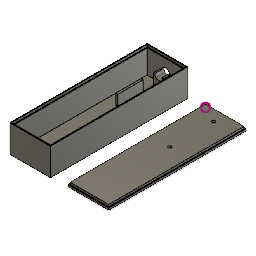
test v3-ok v1 v5 (Autodesk Fusion 360 design; units mm, degrees)
Autodesk Fusion 360 part; units mm, degrees
note: some values were not read from the file. Set by a fixed rule: which face or edge a step refers to.
sketch "スケッチ1" plane through (0, 0, 0) normal (0, 1, 0) x (1, 0, 0)
  line L0 (-40, 10) -> (0, 10)
  line L1 (0, 10) -> (0, -125)
  line L2 (0, -125) -> (-40, -125)
  line L3 (-40, -125) -> (-40, 10)
  line L4 (-31.0482, -10.0567) -> (-29.0482, -10.0567)
  line L5 (-29.0482, -10.0567) -> (-29.0482, -35.0567)
  line L6 (-29.0482, -35.0567) -> (-31.0482, -35.0567)
  line L7 (-31.0482, -35.0567) -> (-31.0482, -10.0567)
  line L8 (-40, -125) -> (-30, -125)
  line L9 (-40, -35) -> (-40, -125)
  line L10 (-40, 10) -> (0, 10)
  line L11 (0, 10) -> (0, 8)
  line L12 (0, 8) -> (-40, 8)
  line L13 (-40, 8) -> (-40, 10)
  line L14 (-40, 10) -> (-38, 10)
  line L15 (-38, 10) -> (-38, -125)
  line L16 (-38, -125) -> (-40, -125)
  line L17 (-40, -125) -> (-40, 10)
  line L18 (0, 10) -> (-2, 10)
  line L19 (-2, 10) -> (-2, -125)
  line L20 (-2, -125) -> (0, -125)
  line L21 (0, -125) -> (0, 10)
  line L22 (-40, -125) -> (0, -125)
  line L23 (0, -125) -> (0, -123)
  line L24 (0, -123) -> (-40, -123)
  line L25 (-40, -123) -> (-40, -125)
  dimension "d1" = 40
  dimension "d2" = 135
  dimension "d3" = 2
  dimension "d4" = 25
  dimension "d5" = 10
  dimension "d6" = 90
  dimension "d7" = 2
  dimension "d8" = 2
  dimension "d9" = 135
  dimension "d10" = 2
  dimension "d11" = 135
  dimension "d12" = 40
  dimension "d13" = 2
  measures "d2" distance of origin
  measures "d4" distance of origin
  measures "d9" distance of origin
  measures "d11" distance of origin
extrude "押し出し1" add sketch "スケッチ1" along normal blind 25 contours L0 L3 L10 L12 L13 L14 L15 L17 | L0 L10 L12 L15 L19 | L3 L9 L12 L15 L17 L24 | L0 L1 L10 L11 L12 L18 L19 L21 | L1 L12 L19 L21 L24 | L2 L8 L15 L19 L22 L24 | L2 L3 L8 L9 L15 L16 L17 L22 L24 L25 | L1 L2 L19 L20 L21 L22 L23 L24 makes body 1
sketch "スケッチ2" plane through (0, 0, 125) normal (0, 0, 1) x (1, 0, 0)
  line L0 (-40, 0) -> (0, 0)
  line L1 (0, 0) -> (0, 25)
  line L2 (0, 25) -> (-40, 25)
  line L3 (-40, 25) -> (-40, 0)
  line L4 (-40, 0) -> (0, 0)
  line L5 (0, 0) -> (0, -2)
  line L6 (0, -2) -> (-40, -2)
  line L7 (-40, -2) -> (-40, 0)
  dimension "d16" = 40
  dimension "d17" = 2
  measures "d17" distance of L0.end
extrude "押し出し2" add sketch "スケッチ2" against normal blind 135 contours L0 L4 L5 L6 L7 bodies 1
sketch "スケッチ3" plane through (0, 0, 0) normal (0, 1, 0) x (1, 0, 0)
  line L0 (-38, -123) -> (-28, -123)
  line L1 (-28, -123) -> (-28, -33)
  line L2 (-28, -33) -> (-38, -33)
  line L3 (-38, -33) -> (-38, -123)
  line L4 (-28, -33) -> (-26, -33)
  line L5 (-26, -33) -> (-26, -8)
  line L6 (-26, -8) -> (-28, -8)
  line L7 (-28, -8) -> (-28, -33)
  dimension "d20" = 90
  dimension "d21" = 10
  dimension "d22" = 25
  dimension "d23" = 2
  measures "d22" distance of origin
extrude "押し出し3" add sketch "スケッチ3" along normal blind 10 contours L4 L5 L6 L7 bodies 1
hole "穴1" at (-20, 11.5, -10) direction (0, 0, 1) diameter 7 depth 15 tip angle 118 bodies 1
sketch "スケッチ4" plane through (0, 0, -10) normal (0, 0, -1) x (-1, 0, 0)
  circle A0 centre (20, 11.5) radius 3.5
  line L0 (40, -2) -> (40, 25)
  line L1 (40, 25) -> (0, 25)
  line L2 (0, 25) -> (0, -2)
  line L3 (0, -2) -> (40, -2)
sketch "スケッチ5" plane through (0, 0, 0) normal (0, 1, 0) x (1, 0, 0)
  line L0 (-24.8616, 8) -> (-15, 8)
  line L1 (-15, 8) -> (-15, -2)
  line L2 (-15, -2) -> (-24.8616, -2)
  line L3 (-24.8616, -2) -> (-24.8616, 8)
  line L4 (-38, 8) -> (-2, 8)
extrude "押し出し4" add sketch "スケッチ5" along normal blind 15 separate body makes body 2
extrude "押し出し5" add 1 faces at (-21.5744, 15, -4.6667) along direction (0, 1, 0) blind 7 on bodies 2 bodies 2 1
extrude "押し出し6" cut sketch "スケッチ4" against normal blind 34 contours A0 bodies 2
extrude "押し出し7" cut 1 faces at (-21.5744, 22, -4.6667) along direction (0, -1, 0) blind 10 on bodies 2 bodies 2
move_face "面をオフセット1" offset -3 1 faces at (-19.8703, 2.6697, 2) on bodies 2
sketch "スケッチ6" plane through (0, 25, 0) normal (0, 1, 0) x (-1, 0, 0)
  line L0 (38, 123) -> (38, -8)
  line L1 (38, -8) -> (2, -8)
  line L2 (2, -8) -> (2, 123)
  line L3 (2, 123) -> (38, 123)
  line L4 (40, -10) -> (40, 125)
  line L5 (40, 125) -> (0, 125)
  line L6 (0, 125) -> (0, -10)
  line L7 (0, -10) -> (40, -10)
  line L8 (39, -9) -> (1, -9)
  line L9 (1, -9) -> (1, 124)
  line L10 (1, 124) -> (39, 124)
  line L11 (39, 124) -> (39, -9)
  dimension "d38" = 133
  measures "d38" distance of origin
extrude "押し出し8" cut sketch "スケッチ6" against normal blind 2 contours L8 L9 L10 L11 bodies 2
sketch "スケッチ7" plane through (0, 0, 0) normal (0, 1, 0) x (1, 0, 0)
  line L0 (18.1709, 9.0329) -> (58.1709, 9.0329)
  line L1 (58.1709, 9.0329) -> (58.1709, -125.9671)
  line L2 (58.1709, -125.9671) -> (18.1709, -125.9671)
  line L3 (18.1709, -125.9671) -> (18.1709, 9.0329)
  dimension "d41" = 135
  dimension "d42" = 40
extrude "押し出し9" add sketch "スケッチ7" along normal blind 2 separate body makes body 3
sketch "スケッチ8" plane through (0, 0, 0) normal (0, 1, 0) x (1, 0, 0)
sketch "スケッチ9" plane through (0, 2, 0) normal (0, 1, 0) x (-1, 0, 0)
  line L0 (-18.1709, 125.9671) -> (-58.1709, 125.9671)
  line L1 (-58.1709, 125.9671) -> (-58.1709, -9.0329)
  line L2 (-58.1709, -9.0329) -> (-18.1709, -9.0329)
  line L3 (-18.1709, -9.0329) -> (-18.1709, 125.9671)
  line L4 (-18.1709, -9.0329) -> (-19.1709, -9.0329)
  line L5 (-19.1709, -9.0329) -> (-19.1709, -8.0329)
  line L6 (-19.1709, -8.0329) -> (-18.1709, -8.0329)
  line L7 (-18.1709, -8.0329) -> (-18.1709, -9.0329)
  line L8 (-19.1709, -8.0329) -> (-57.1709, -8.0329)
  line L9 (-57.1709, -8.0329) -> (-57.1709, 124.9671)
  line L10 (-57.1709, 124.9671) -> (-19.1709, 124.9671)
  line L11 (-19.1709, 124.9671) -> (-19.1709, -8.0329)
  dimension "d45" = 1
  dimension "d46" = 1
  dimension "d47" = 38
  dimension "d48" = 133
extrude "押し出し10" add sketch "スケッチ9" along normal blind 2 contours L8 L9 L10 L11 bodies 3
form "フォーム1" [no effect]
sketch "スケッチ10" plane through (0, 0, 0) normal (0, 1, 0) x (1, 0, 0)
hole "穴2" at (38.1729, 4, 2.9601) direction (0, -1, 0) diameter 3 depth 32.5 tip angle 118 bodies 3
sketch "スケッチ11" plane through (0, 0, 0) normal (0, 1, 0) x (1, 0, 0)
hole "穴3" at (38.1698, 4, 45.9669) direction (0, -1, 0) diameter 2 depth 12.5 tip angle 118 bodies 3
sketch "スケッチ12" plane through (-40, 0, 0) normal (-1, 0, 0) x (0, 0, 1)
  line L0 (125, -2) -> (125, 25)
  line L1 (125, 25) -> (-10, 25)
  line L2 (-10, 25) -> (-10, -2)
  line L3 (-10, -2) -> (125, -2)
  line L4 (5.8366, 7.0992) -> (72.8561, 7.0992) construction
  line L5 (72.8561, 7.0992) -> (72.8561, 19.0992) construction
  line L6 (72.8561, 19.0992) -> (5.8366, 19.0992) construction
  line L7 (5.8366, 19.0992) -> (5.8366, 7.0992) construction
  text T0 "SecHack365" font "Arial" height 12 align ink ink in box 0 x 0 at (5.8366, 7.0992) x (1, 0) y (0, 1) spacing 1 height is em
extrude "押し出し11" cut sketch "スケッチ12" against normal blind 1 text T0 bodies 2
hole "穴4" at (38.1698, 4, 45.9669) direction (0, -1, 0) diameter 3 depth 7.5 tip angle 118 bodies 3
extrude "押し出し12" add 1 faces at (-39, 11.3872, 9.9712) along direction (-1, 0, 0) blind 0.5 on bodies 2 bodies 2
extrude "押し出し13" add 9 faces at (-39, 10.4024, 17.5653) (-39, 8.5001, 21.2893) (-39, 11.4845, 33.3056) (-39, 9.0381, 40.1197) (-39, 8.5001, 42.6291) (-39, 11.3653, 48.4735) (-39, 11.9074, 57.3496) (-39, 11.8533, 60.8192) (-39, 15.4083, 69.8954) along direction (-1, 0, 0) blind 0.5 on bodies 2 bodies 2
